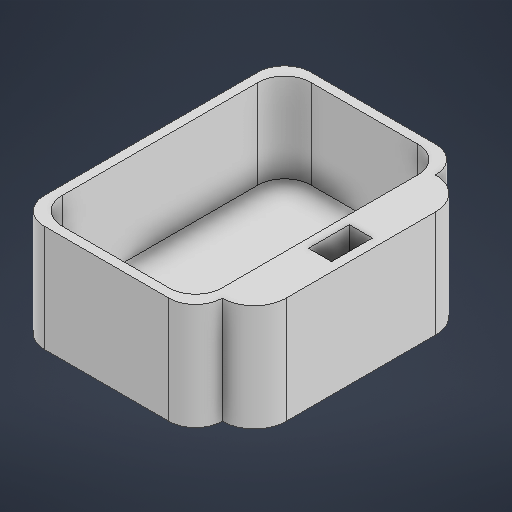
# Autodesk Inventor part: box
Saved by Autodesk Inventor 2026 (Build 300175050, 175E)
## iProperties
Created: 2025-05-28
Part Number: box
Material: Generic
Document SubType Name: Modeling
Designer: niall
Density: 1 g/cm^3
Appearance: Default
Author: niall
Autodesk Inventor part; units mm, degrees
ref_plane "YZ Plane" through (0, 0, 0) normal (1, 0, 0) x (0, 1, 0)
ref_plane "XZ Plane" through (0, 0, 0) normal (0, 1, 0) x (-1, 0, 0)
ref_plane "XY Plane" through (0, 0, 0) normal (0, 0, 1) x (1, 0, 0)
sketch "Sketch1" plane through (0, 0, 0) normal (0, 1, 0) x (-1, 0, 0)
  line L0 (-50, -75) -> (50, -75)
  line L1 (50, -75) -> (50, 75)
  line L2 (50, 75) -> (-50, 75)
  line L3 (-50, 75) -> (-50, -75)
  line L4 (-50, -75) -> (50, 75) construction
  line L5 (50, -75) -> (-50, 75) construction
  point P0 (0, 0)
  dimension "d0" = 100
  dimension "d1" = 150
  constraints: 12 end point, 2 midpoint, 2 parallel, 1 horizontal, 1 perpendicular
  measures "d0" distance of L2.end L1.end
  measures "d1" distance of L1.end L0.end
extrude "Extrusion1" add sketch "Sketch1" along normal blind 60
sketch "Sketch2" plane through (0, 60, 0) normal (0, 1, 0) x (1, 0, 0)
  line L0 (45, 70) -> (-45, 70)
  line L1 (-45, 70) -> (-45, -70)
  line L2 (-45, -70) -> (45, -70)
  line L3 (45, -70) -> (45, 70)
  line L4 (45, 70) -> (-45, -70) construction
  line L5 (-45, 70) -> (45, -70) construction
  point P0 (0, 0)
  dimension "d4" = 90
  dimension "d5" = 140
  constraints: 12 end point, 2 midpoint, 2 parallel, 1 horizontal, 1 perpendicular
  measures "d4" distance of L2.end L1.end
  measures "d5" distance of L1.end L0.end
extrude "Extrusion2" cut sketch "Sketch2" against normal blind 50
fillet "Fillet1" radius 15 8 edges at (-45, 35, 70) (-45, 35, -70) (45, 35, -70) (45, 35, 70) (50, 30, 75) (-50, 30, 75) (50, 30, -75) (-50, 30, -75)
sketch "Sketch3" plane through (50, 0, 60) normal (1, 0, 0) x (0, 0, -1)
  line L0 (0, 60) -> (0, 0) projected
  line L1 (0, 0) -> (120, 0) projected
  line L2 (0, 60) -> (120, 60)
  line L3 (120, 60) -> (120, 0)
  line L4 (120, 0) -> (0, 0)
  line L5 (0, 0) -> (0, 60)
  point P0 (60, 0)
  constraints: 8 end point, 2 parallel, 1 horizontal, 1 perpendicular
extrude "Extrusion3" add sketch "Sketch3" along normal blind 18
fillet "Fillet2" radius 18 2 edges at (68, 30, 60) (68, 30, -60)
sketch "Sketch4" plane through (0, 60, 0) normal (0, 1, 0) x (1, 0, 0)
  arc A0 (68, 42) -> (50, 60) centre (50, 42) ccw projected
  line L0 (50, -60) -> (50, 60)
  line L1 (50, 0) -> (63, 0)
  line L2 (63, 0) -> (63, 11.5)
  line L3 (63, 11.5) -> (50, 11.5)
  line L4 (50, 11.5) -> (50, 0)
  line L5 (50, 0) -> (63, 0)
  line L6 (63, 0) -> (63, -11.5)
  line L7 (63, -11.5) -> (50, -11.5)
  line L8 (50, -11.5) -> (50, 0)
  point P0 (0, 0)
  dimension "d12" = 13
  dimension "d13" = 11.5
  dimension "d14" = 11.5
  constraints: 18 end point, 4 parallel, 2 horizontal, 2 perpendicular, 1 midpoint, 1 point on line, 1 vertical
  measures "d12" distance of L3.end L2.end
  measures "d13" distance of L2.end L1.end
  measures "d14" distance of L5.end L6.end
extrude "Extrusion4" cut sketch "Sketch4" against normal blind 25
body "Solid1"
